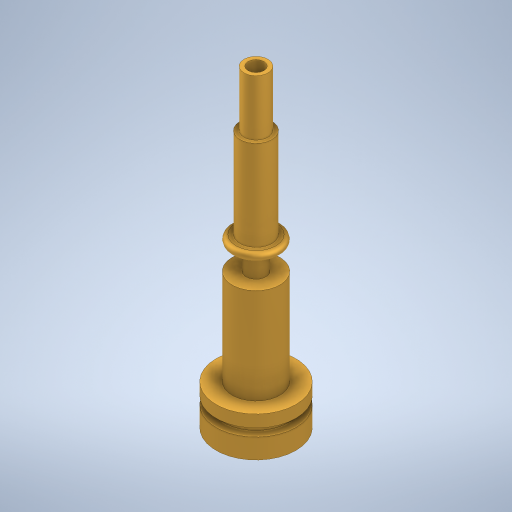
# Autodesk Inventor part: Revo micro nozzle
Saved by Autodesk Inventor 2023.1 (Build 271208000, 208)
## iProperties
Created: 2022-11-20
Part Number: Revo micro nozzle
Material: Brass, Soft Yellow
Document SubType Name: Modeling
Designer: Frank
Mass: 7.00139 g
Surface Area: 11.3734 cm^2
Volume: 0.82661 cm^3
Density: 8.47 g/cm^3
Appearance: Brass - Satin
Author: Frank
Autodesk Inventor part; units mm, degrees
ref_plane "YZ Plane" through (0, 0, 0) normal (1, 0, 0) x (0, 1, 0)
ref_plane "XZ Plane" through (0, 0, 0) normal (0, 1, 0) x (-1, 0, 0)
ref_plane "XY Plane" through (0, 0, 0) normal (0, 0, 1) x (1, 0, 0)
sketch "Sketch1" plane through (0, 0, 0) normal (0, 0, 1) x (1, 0, 0)
  line L0 (0, 20.65) -> (0, -20.65)
  line L1 (0, 1.35) -> (-2.5, 1.35)
  arc A0 (-2.5, 2.35) -> (-2.5, 1.35) centre (-2.5, 1.85) ccw
  line L2 (-2.5, 2.35) -> (0, 2.35)
  line L3 (-0.3, -20.65) -> (-0.8453, -20.65)
  line L4 (-0.8453, -20.65) -> (-2, -18.65)
  line L5 (-2, -18.65) -> (-5, -18.65)
  line L6 (-0.3, -20.65) -> (-1, -16.6801)
  line L7 (-1, -16.6801) -> (-1, 20.65)
  line L8 (-1.25, 1.35) -> (-1.25, -1.65)
  line L9 (-1.25, -1.65) -> (-3, -1.65)
  line L10 (-3, -1.65) -> (-3, -13.65)
  line L11 (-3, -13.65) -> (-5, -13.65)
  line L12 (-5, -13.65) -> (-5, -15.15)
  line L13 (-5, -15.15) -> (-4, -15.15)
  line L14 (-4, -15.15) -> (-4, -16.15)
  line L15 (-4, -16.15) -> (-5, -16.15)
  line L16 (-5, -16.15) -> (-5, -18.65)
  line L17 (-5, -13.65) -> (-5, -18.65) construction
  line L18 (-2, 2.35) -> (-2, 13.65)
  line L19 (-2, 13.65) -> (-1.5, 13.65)
  line L20 (-1.5, 13.65) -> (-1.5, 20.65)
  line L21 (-1.5, 20.65) -> (0, 20.65)
  point P0 (0, 0)
  point P1 (0, 0)
  dimension "d0" = 41.3
  dimension "d1" = 21
  dimension "d2" = 2
  dimension "d3" = 2
  dimension "d4" = 0.6
  dimension "d5" = 10
  dimension "d6" = 4
  dimension "d7" = 60
  dimension "d8" = 10
  dimension "d9" = 1
  dimension "d10" = 5
  dimension "d11" = 2.5
  dimension "d12" = 5
  dimension "d13" = 12
  dimension "d14" = 6
  dimension "d15" = 1
  dimension "d16" = 1.5
  dimension "d17" = 3
  dimension "d18" = 4
  dimension "d19" = 7
  constraints: 44 end point, 13 perpendicular, 5 point on line, 4 vertical, 3 horizontal, 2 midpoint, 2 point on circle, 2 tangent, 1 centre point, 1 coincident, 1 horizontal alignment, 1 parallel
  measures "d0" distance of L0.start L0.end
  measures "d1" distance between parallel lines of L5 L2
  measures "d2" distance from line of L5 L0.end
  measures "d3" diameter of L7 L0
  measures "d4" diameter of L3.start L0
  measures "d5" diameter of L5.end L0
  measures "d6" diameter of L4.end L0
  measures "d7" angle of L5 L4
  measures "d8" angle of L0 L6
  measures "d9" distance between parallel lines of L2 L1
  measures "d10" diameter of A0.centre L0
  measures "d11" diameter of L8 L0
  measures "d12" distance between parallel lines of L5 L11
  measures "d13" distance of L9.end L10.end
  measures "d14" diameter of L10 L0
  measures "d15" distance of L13.end L14.end
  measures "d16" distance between parallel lines of L11 L13
  measures "d17" diameter of L20 L0
  measures "d18" diameter of L18 L0
  measures "d19" distance between parallel lines of L21 L19
revolve "Revolution1" add sketch "Sketch1" angle 360 about axis through (0, 20.65, 0) along (0, -1, 0) contours L7 L2 L18 L19 L20 L21 | L7 L1 A0 L2 | L7 L6 L3 L4 L5 L16 L15 L14 L13 L12 L11 L10 L9 L8 L1
body "Solid1"
